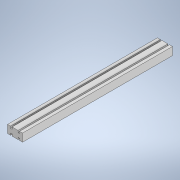
# Autodesk Inventor part: Linear Rail Base
Saved by Autodesk Inventor 2022 (Build 260153000, 153)
## iProperties
Created: 2021-11-30
Part Number: Linear Rail Base
Material: Generic
Document SubType Name: Modeling
Designer: efred
Density: 1 g/cm^3
Appearance: Default
Author: efred
Autodesk Inventor part; units mm, degrees
ref_plane "YZ Plane" through (0, 0, 0) normal (1, 0, 0) x (0, 1, 0)
ref_plane "XZ Plane" through (0, 0, 0) normal (0, 1, 0) x (-1, 0, 0)
ref_plane "XY Plane" through (0, 0, 0) normal (0, 0, 1) x (1, 0, 0)
sketch "Sketch1" plane through (0, 0, 0) normal (0, 1, 0) x (-1, 0, 0)
  line L0 (-19.95, 199) -> (19.95, 199)
  line L1 (19.95, 199) -> (19.95, -199)
  line L2 (19.95, -199) -> (-19.95, -199)
  line L3 (-19.95, -199) -> (-19.95, 199)
  line L4 (-19.95, 199) -> (19.95, -199) construction
  line L5 (19.95, 199) -> (-19.95, -199) construction
  point P0 (0, 0)
  dimension "d0" = 39.9
  dimension "d1" = 398
  constraints: 12 end point, 2 midpoint, 2 parallel, 1 horizontal, 1 perpendicular
  measures "d0" distance between parallel lines of L3 L1
  measures "d1" distance between parallel lines of L0 L2
extrude "Extrusion1" add sketch "Sketch1" along normal mid plane 21
sketch "Sketch2" plane through (0, 10.5, 0) normal (0, 1, 0) x (1, 0, 0)
  line L0 (-19.95, -199) -> (19.95, -199) projected
  line L1 (19.95, 199) -> (-19.95, 199) projected
  line L2 (-11.95, -199) -> (-7.95, -199)
  line L3 (-7.95, -199) -> (-7.95, 199)
  line L4 (-7.95, 199) -> (-11.95, 199)
  line L5 (-11.95, 199) -> (-11.95, -199)
  line L6 (0, -199) -> (0, 199) construction
  line L7 (-19.95, 199) -> (-19.95, -199) projected
  line L8 (7.95, -199) -> (11.95, -199)
  line L9 (11.95, -199) -> (11.95, 199)
  line L10 (11.95, 199) -> (7.95, 199)
  line L11 (7.95, 199) -> (7.95, -199)
  point P0 (0, 0)
  point P1 (-11.95, 199)
  dimension "d4" = 4
  dimension "d5" = 8
  constraints: 18 end point, 4 parallel, 4 point on line, 2 horizontal, 2 midpoint, 2 perpendicular, 2 other
  measures "d4" distance between parallel lines of L3 L5
  measures "d5" distance between parallel lines of L7 L5
extrude "Extrusion2" cut sketch "Sketch2" against normal blind 5 contours L5 L1 L3 L0 | L11 L1 L9 L0
mirror "Mirror1" about plane through (0, 0, 0) normal (0, 1, 0) of "Extrusion2"
body "Solid1"
